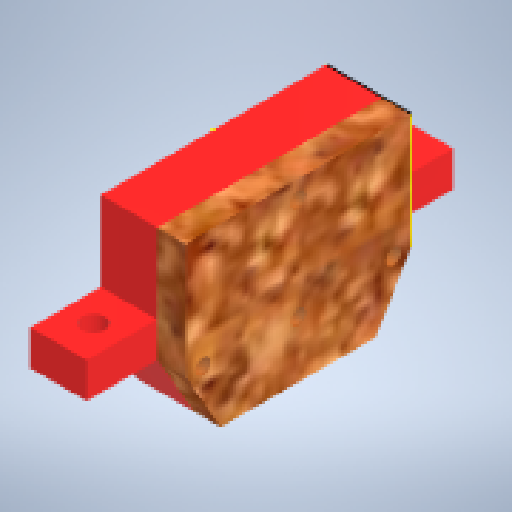
# Autodesk Inventor part: Det_podsh
Saved by Autodesk Inventor 2023.1 (Build 271208000, 208)
## iProperties
Created: 2023-12-24
Part Number: Det_podsh
Material: Типовые
Document SubType Name: Modeling
Designer: Dell
Density: 1 g/cm^3
Appearance: По умолчанию
Author: Dell
Autodesk Inventor part; units mm, degrees
ref_plane "XZ Plane" through (0, 0, 0) normal (0, 1, 0) x (-1, 0, 0)
ref_plane "XY Plane" through (0, 0, 0) normal (0, 0, 1) x (1, 0, 0)
sketch "Эскиз1" plane through (0, 0, 0) normal (1, 0, 0) x (0, 1, 0)
  line L0 (25, 0) -> (25, -32)
  line L1 (0, 0) -> (12.5, 5)
  line L2 (12.5, 5) -> (25, 0)
  line L3 (0, -32) -> (15.6161, -32.8571)
  line L4 (15.6161, -32.8571) -> (25, -32)
  line L5 (0, -16) -> (25, -16) construction
  arc A0 (0, -24.2614) -> (0, -7.7386) centre (8, -16) ccw
  line L6 (0, -32) -> (0, -24.2614)
  line L7 (0, -7.7386) -> (0, 0)
  circle A1 centre (8, -16) radius 4.5
  point P0 (12.5, 0)
  point P1 (10.7952, -31.5311)
  point P2 (0, -5)
  point P3 (0, -27)
  dimension "d10" = 5
  dimension "d11" = 5
  dimension "d12" = 5
  dimension "d13" = 5
  dimension "d14" = 8
  dimension "d15" = 23
  dimension "d16" = 9
  constraints: 16 end point, 3 point on line, 2 centre point, 2 coincident, 2 parallel, 2 point on circle, 1 midpoint
  measures "d10" distance of point (12.5, 0) L1.end
  measures "d11" distance of point (10.795, -31.531) L3.end
  measures "d12" distance of L1.start point (0, -5)
  measures "d13" distance of point (0, -27) L3.start
  measures "d14" distance of point (0, -16) point (8, -16)
  measures "d15" diameter of A0
  measures "d16" diameter of A1
sketch "Эскиз2" plane through (0, 0, 0) normal (1, 0, 0) x (0, 1, 0)
  line L0 (-12.5, -16) -> (12.5, -16) construction
  line L1 (12.5, -16) -> (12.5, 16)
  line L2 (12.5, 16) -> (-12.5, 16) construction
  line L3 (-12.5, 16) -> (-12.5, -16) construction
  line L4 (-12.5, -16) -> (12.5, 16) construction
  line L5 (12.5, -16) -> (-12.5, 16) construction
  line L6 (0, 0) -> (47.464, 0) construction
  line L7 (-3.8397, 16) -> (-12.5, 11)
  line L8 (-3.8397, -16) -> (-12.5, -11)
  line L9 (-12.5, 11) -> (-12.5, -11)
  line L10 (-3.8397, -16) -> (12.5, -16)
  line L11 (-3.8397, 16) -> (12.5, 16)
  dimension "d17" = 32
  dimension "d18" = 30
  dimension "d19" = 25
  dimension "d20" = 22
  constraints: 24 end point, 2 collinear, 2 horizontal, 2 midpoint, 2 parallel, 2 perpendicular, 2 point on line, 2 symmetric about line
  measures "d17" distance of L0.end L1.end
  measures "d18" angle of L2 L7
  measures "d19" distance between parallel lines of L3 L1
  measures "d20" distance of L8.end L7.end
extrude "Выдавливание1" add sketch "Эскиз2" along normal blind 8
extrude "Выдавливание3" add sketch "Эскиз2" along normal blind 4 from surface at 8 separate body
sketch "Эскиз3" plane through (8, 0, 0) normal (1, 0, 0) x (0, 0, -1)
  line L0 (-11, -12.5) -> (11, -12.5) construction
  line L1 (0, -12.5) -> (0, 14.5012) construction
  circle A0 centre (0, -4.5) radius 4.75
  circle A1 centre (0, -4.5) radius 11.25
  point P0 (0, 0)
  dimension "d23" = 22.5
  dimension "d24" = 9.5
  dimension "d25" = 8
  constraints: 2 centre point, 2 end point, 1 coincident, 1 midpoint, 1 point on line, 1 vertical
  measures "d23" diameter of A1
  measures "d24" diameter of A0
  measures "d25" distance from line of L0 A0.centre
extrude "Выдавливание2" cut sketch "Эскиз3" against normal blind 6.3 bodies 1
sketch "Эскиз4" plane through (1.7, 0, 0) normal (1, 0, 0) x (0, 0, -1)
  circle A0 centre (0, -4.5) radius 4.75 projected
  circle A1 centre (0, -4.5) radius 6.5
  point P0 (0, 0)
  dimension "d30" = 13
  constraints: 1 centre point
  measures "d30" diameter of A1
extrude "Выдавливание4" add sketch "Эскиз4" along normal blind 0.3 bodies 1
sketch "Эскиз5" plane through (0, 0, 0) normal (0, 0, 1) x (1, 0, 0)
  line L0 (2, 0.25) -> (8, 0.25) projected
  line L1 (2, -11) -> (2, 2) projected
  line L2 (2, 0.45) -> (6.8, 0.45)
  line L3 (6.8, 0.45) -> (7, 0.25)
  line L4 (8, -9.25) -> (8, 0.25) projected
  line L5 (8, -4.5) -> (11.75, -4.5)
  point P0 (0, 0)
  dimension "d33" = 0.2
  dimension "d34" = 135
  dimension "d35" = 1
  constraints: 6 end point, 2 point on line, 1 horizontal, 1 midpoint
  measures "d33" distance between parallel lines of L2 L0
  measures "d34" angle of L2 L3
  measures "d35" distance of L3.end L0.end
revolve "Вращение1" add sketch "Эскиз5" angle 15 mid plane about axis through (8, -4.5, 0) along (1, 0, 0) bodies 1
ref_plane "РабПлоскость2" through (4, 12.5, -16) normal (1, 0, 0) x (0, 0, -1)
ref_plane "РабПлоскость1" through (8, 12.5, -16) normal (1, 0, 0) x (0, 0, -1)
sketch "Эскиз6" plane through (4, 12.5, -16) normal (1, 0, 0) x (0, 0, -1)
  point P0 (-16, -12.5)
pattern_circular "Круговой массив1" count 12 over 360 about axis through (8, -4.5, 0) along (-1, 0, 0) of "Вращение1" bodies 1
sketch "Эскиз8" plane through (12, -3.8397, -16) normal (1, 0, 0) x (0, 0, -1)
  line L0 (-32, 0) -> (-27, -8.6603) projected
  line L1 (-5, -8.6603) -> (0, 0) projected
  line L2 (-32, 0) -> (0, 0) construction
  circle A0 centre (-29.5, 0) radius 1.1
  circle A1 centre (-2.5, 0) radius 1.1
  circle A2 centre (-16, 13.782) radius 1.1
  circle A3 centre (-16, -0.6603) radius 4.75 projected
  circle A4 centre (-16, -0.6603) radius 1.1
  point P0 (-16, 3.8397)
  dimension "d40" = 2.2
  dimension "d41" = 2.2
  dimension "d42" = 2.2
  dimension "d47" = 2.2
  constraints: 4 centre point, 2 end point, 2 point on line, 1 coincident, 1 horizontal
  measures "d40" diameter of A0
  measures "d41" diameter of A1
  measures "d42" diameter of A2
  measures "d47" diameter of A4
extrude "Выдавливание6" cut sketch "Эскиз8" against normal blind 8.5 contours A0 | A1 | A2 | A4 bodies 2 1
sketch "Эскиз9" plane through (0, 12.5, 16) normal (0, 1, 0) x (1, 0, 0)
  point P0 (0, 16)
sketch "Эскиз10" plane through (0, -3.8397, -16) normal (0, 0, -1) x (-1, 0, 0)
  line L0 (0, 16.3397) -> (0, 0) projected
  line L1 (0, 5.0414) -> (-8, 5.0414)
  line L2 (-8, 5.0414) -> (-8, 0.0414)
  line L3 (-8, 0.0414) -> (0, 0.0414)
  line L4 (0, 0.0414) -> (0, 5.0414)
  point P0 (0, 3.8397)
  dimension "d49" = 8
  dimension "d50" = 5
  constraints: 8 end point, 2 parallel, 1 horizontal, 1 perpendicular, 1 point on line
  measures "d49" distance of L3.end L2.end
  measures "d50" distance of L2.end L1.end
extrude "Выдавливание7" add sketch "Эскиз10" along normal blind 10 bodies 1
sketch "Эскиз13" plane through (0, -3.7984, -16) normal (0, -1, 0) x (1, 0, 0)
  line L0 (8, -10) -> (0, -10) projected
  line L1 (0, -10) -> (8, 0) construction
  line L2 (0, 0) -> (8, 0) projected
  line L3 (8, 0) -> (8, -10) projected
  line L4 (0, 0) -> (8, -10) construction
  line L5 (4, -8.262) -> (1.175, -6.631)
  line L6 (1.175, -6.631) -> (1.175, -3.369)
  line L7 (1.175, -3.369) -> (4, -1.738)
  line L8 (4, -1.738) -> (6.825, -3.369)
  line L9 (6.825, -3.369) -> (6.825, -6.631)
  line L10 (6.825, -6.631) -> (4, -8.262)
  point P0 (0, 16)
  point P1 (4, -5)
  point P2 (6.825, -5)
  point P3 (1.175, -5)
  dimension "d60" = 5.65
  constraints: 16 end point, 3 midpoint, 13 other
  measures "d60" distance of point (6.825, -5) point (1.175, -5)
extrude "Выдавливание10" cut sketch "Эскиз13" against normal blind 2.45 bodies 1
sketch "Эскиз14" plane through (0, -1.3484, -16) normal (0, -1, 0) x (1, 0, 0)
  line L0 (1.175, -6.631) -> (1.175, -3.369) projected
  line L1 (1.175, -6.631) -> (6.7033, -3.369) construction
  line L2 (6.7033, -3.369) -> (1.175, -3.369) construction
  line L3 (1.175, -3.369) -> (6.7033, -6.631) construction
  circle A0 centre (3.9391, -5) radius 1.65
  point P0 (0, 16)
  dimension "d63" = 3.3
  constraints: 6 end point, 1 centre point, 1 midpoint, 1 perpendicular
  measures "d63" diameter of A0
extrude "Выдавливание11" cut sketch "Эскиз14" against normal blind 10 bodies 1
mirror "Зеркальное отражение2" about plane through (0, 0, 0) normal (0, 0, 1) of "Выдавливание10", "Выдавливание7", "Выдавливание11" bodies 1
sketch "Эскиз15" plane through (8, 12.5, -16) normal (0, 0, -1) x (-1, 0, 0)
  line L0 (-4, -16.3397) -> (-4, 0) projected
  line L1 (8, 0) -> (0, 0) projected
  line L2 (-4, 0) -> (8, 0)
  point P0 (8, -12.5)
  constraints: 2 end point, 1 collinear
sketch "Эскиз16" plane through (8, -3.8397, -16) normal (-1, 0, 0) x (0, 0, 1)
  circle A0 centre (16, -0.6603) radius 11 construction
  circle A1 centre (16, -0.6603) radius 5 construction
  circle A2 centre (16, -0.6603) radius 1.1 projected
  circle A3 centre (16, -0.6603) radius 11.25
  point P0 (16, 3.8397)
  dimension "d66" = 22
  dimension "d67" = 22.5
  constraints: 1 centre point, 1 coincident
  measures "d66" diameter of A0
  measures "d67" diameter of A3
extrude "Выдавливание12" cut sketch "Эскиз16" against normal blind 2 bodies 2
